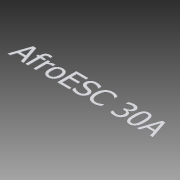
# Autodesk Inventor part: afro
Saved by Autodesk Inventor 2012 (Build 160160000, 160)
## iProperties
Created: 2014-07-18
Part Number: afro
Material: Default
Document SubType Name: Modeling
Designer: Anon
Density: 1 g/cm^3
Author: Anon
Autodesk Inventor part; units mm, degrees
ref_plane "YZ Plane" through (0, 0, 0) normal (1, 0, 0) x (0, 1, 0)
ref_plane "XZ Plane" through (0, 0, 0) normal (0, 1, 0) x (-1, 0, 0)
ref_plane "XY Plane" through (0, 0, 0) normal (0, 0, 1) x (1, 0, 0)
sketch "Sketch1" plane through (0, 0, 0) normal (0, 0, 1) x (1, 0, 0)
  line L0 (-5.9322, 2.9237) -> (28.5593, 2.9237) construction
  line L1 (28.5593, 2.9237) -> (28.5593, -13.2627) construction
  line L2 (28.5593, -13.2627) -> (-5.9322, -13.2627) construction
  line L3 (-5.9322, -13.2627) -> (-5.9322, 2.9237) construction
  line L4 (-5.9549, -0.755) -> (-4.775, 2.745)
  line L5 (-4.775, 2.745) -> (-4.2021, 2.745)
  line L6 (-4.2021, 2.745) -> (-3.0222, -0.755)
  line L7 (-3.0222, -0.755) -> (-3.5128, -0.755)
  line L8 (-3.5128, -0.755) -> (-3.8305, 0.2236)
  line L9 (-3.8305, 0.2236) -> (-5.1664, 0.2236)
  line L10 (-5.1664, 0.2236) -> (-5.4841, -0.755)
  line L11 (-5.4841, -0.755) -> (-5.9549, -0.755)
  line L12 (-3.9581, 0.6206) -> (-4.4999, 2.2685)
  line L13 (-4.4999, 2.2685) -> (-5.0388, 0.6206)
  line L14 (-5.0388, 0.6206) -> (-3.9581, 0.6206)
  line L15 (-1.3431, 2.4756) -> (-1.3658, 2.4756)
  spline S0 degree 2 poles (-1.3658, 2.4756) (-1.4253, 2.4983) (-1.6465, 2.538) (-1.7345, 2.538) knots 0 0 0 1 2 2 2
  spline S1 degree 2 poles (-1.7345, 2.538) (-2.0124, 2.538) (-2.2507, 2.2884) (-2.2507, 1.9594) knots 0 0 0 1 2 2 2
  line L16 (-2.2507, 1.9594) -> (-2.2507, 1.8715)
  line L17 (-2.2507, 1.8715) -> (-1.5189, 1.8715)
  line L18 (-1.5189, 1.8715) -> (-1.5189, 1.5056)
  line L19 (-1.5189, 1.5056) -> (-2.2365, 1.5056)
  line L20 (-2.2365, 1.5056) -> (-2.2365, -0.755)
  line L21 (-2.2365, -0.755) -> (-2.679, -0.755)
  line L22 (-2.679, -0.755) -> (-2.679, 1.5056)
  line L23 (-2.679, 1.5056) -> (-2.9768, 1.5056)
  line L24 (-2.9768, 1.5056) -> (-2.9768, 1.8715)
  line L25 (-2.9768, 1.8715) -> (-2.679, 1.8715)
  line L26 (-2.679, 1.8715) -> (-2.679, 1.9594)
  spline S2 degree 2 poles (-2.679, 1.9594) (-2.679, 2.4302) (-2.2223, 2.9237) (-1.7969, 2.9237) knots 0 0 0 1 2 2 2
  spline S3 degree 2 poles (-1.7969, 2.9237) (-1.6749, 2.9237) (-1.4395, 2.8982) (-1.3431, 2.8812) knots 0 0 0 1 2 2 2
  line L27 (-1.3431, 2.8812) -> (-1.3431, 2.4756)
  line L28 (0.1999, 1.3978) -> (0.1772, 1.3978)
  spline S4 degree 2 poles (0.1772, 1.3978) (0.1261, 1.412) (0.0155, 1.4177) (-0.0611, 1.4177) knots 0 0 0 1 2 2 2
  spline S5 degree 2 poles (-0.0611, 1.4177) (-0.2397, 1.4177) (-0.5914, 1.2617) (-0.7503, 1.1085) knots 0 0 0 1 2 2 2
  line L29 (-0.7503, 1.1085) -> (-0.7503, -0.755)
  line L30 (-0.7503, -0.755) -> (-1.1927, -0.755)
  line L31 (-1.1927, -0.755) -> (-1.1927, 1.8715)
  line L32 (-1.1927, 1.8715) -> (-0.7503, 1.8715)
  line L33 (-0.7503, 1.8715) -> (-0.7503, 1.48)
  spline S6 degree 2 poles (-0.7503, 1.48) (-0.5092, 1.6956) (-0.149, 1.8715) (0.0212, 1.8715) knots 0 0 0 1 2 2 2
  spline S7 degree 2 poles (0.0212, 1.8715) (0.0893, 1.8715) (0.1573, 1.8658) (0.1999, 1.8573) knots 0 0 0 1 2 2 2
  line L34 (0.1999, 1.8573) -> (0.1999, 1.3978)
  spline S8 degree 2 poles (2.7015, 0.5583) (2.7015, -0.1054) (2.0633, -0.8287) (1.5301, -0.8287) knots 0 0 0 1 2 2 2
  spline S9 degree 2 poles (1.5301, -0.8287) (0.9827, -0.8287) (0.3559, -0.0828) (0.3559, 0.5583) knots 0 0 0 1 2 2 2
  spline S10 degree 2 poles (0.3559, 0.5583) (0.3559, 1.2163) (1.0026, 1.9452) (1.5301, 1.9452) knots 0 0 0 1 2 2 2
  spline S11 degree 2 poles (1.5301, 1.9452) (2.0633, 1.9452) (2.7015, 1.2191) (2.7015, 0.5583) knots 0 0 0 1 2 2 2
  spline S12 degree 2 poles (2.2449, 0.5583) (2.2449, 1.0688) (1.8733, 1.5651) (1.5301, 1.5651) knots 0 0 0 1 2 2 2
  spline S13 degree 2 poles (1.5301, 1.5651) (1.1869, 1.5651) (0.8125, 1.0688) (0.8125, 0.5583) knots 0 0 0 1 2 2 2
  spline S14 degree 2 poles (0.8125, 0.5583) (0.8125, 0.0619) (1.1869, -0.4486) (1.5301, -0.4486) knots 0 0 0 1 2 2 2
  spline S15 degree 2 poles (1.5301, -0.4486) (1.8705, -0.4486) (2.2449, 0.0534) (2.2449, 0.5583) knots 0 0 0 1 2 2 2
  line L35 (3.1894, -0.755) -> (3.1894, 2.745)
  line L36 (3.1894, 2.745) -> (5.379, 2.745)
  line L37 (5.379, 2.745) -> (5.379, 2.3309)
  line L38 (5.379, 2.3309) -> (3.6545, 2.3309)
  line L39 (3.6545, 2.3309) -> (3.6545, 1.3723)
  line L40 (3.6545, 1.3723) -> (5.2627, 1.3723)
  line L41 (5.2627, 1.3723) -> (5.2627, 0.9582)
  line L42 (5.2627, 0.9582) -> (3.6545, 0.9582)
  line L43 (3.6545, 0.9582) -> (3.6545, -0.3409)
  line L44 (3.6545, -0.3409) -> (5.379, -0.3409)
  line L45 (5.379, -0.3409) -> (5.379, -0.755)
  line L46 (5.379, -0.755) -> (3.1894, -0.755)
  spline S16 degree 2 poles (6.8652, -0.8174) (6.4851, -0.8174) (5.9519, -0.6585) (5.7165, -0.5451) knots 0 0 0 1 2 2 2
  line L47 (5.7165, -0.5451) -> (5.7165, 0.0392)
  line L48 (5.7165, 0.0392) -> (5.7505, 0.0392)
  spline S17 degree 2 poles (5.7505, 0.0392) (5.9803, -0.1764) (6.5617, -0.4146) (6.8312, -0.4146) knots 0 0 0 1 2 2 2
  spline S18 degree 2 poles (6.8312, -0.4146) (7.2169, -0.4146) (7.6112, -0.0941) (7.6112, 0.1697) knots 0 0 0 1 2 2 2
  spline S19 degree 2 poles (7.6112, 0.1697) (7.6112, 0.3796) (7.4041, 0.6405) (7.18, 0.7057) knots 0 0 0 1 2 2 2
  spline S20 degree 2 poles (7.18, 0.7057) (7.0184, 0.7511) (6.7489, 0.8135) (6.5475, 0.8646) knots 0 0 0 1 2 2 2
  spline S21 degree 2 poles (6.5475, 0.8646) (6.366, 0.9128) (6.0795, 1.0574) (5.9689, 1.1737) knots 0 0 0 1 2 2 2
  spline S22 degree 2 poles (5.9689, 1.1737) (5.8612, 1.29) (5.742, 1.602) (5.742, 1.8062) knots 0 0 0 1 2 2 2
  spline S23 degree 2 poles (5.742, 1.8062) (5.742, 2.2317) (6.4057, 2.8074) (6.9191, 2.8074) knots 0 0 0 1 2 2 2
  spline S24 degree 2 poles (6.9191, 2.8074) (7.2141, 2.8074) (7.7359, 2.6912) (7.96, 2.5805) knots 0 0 0 1 2 2 2
  line L49 (7.96, 2.5805) -> (7.96, 2.0246)
  line L50 (7.96, 2.0246) -> (7.926, 2.0246)
  spline S25 degree 2 poles (7.926, 2.0246) (7.7586, 2.1778) (7.2368, 2.4047) (6.9503, 2.4047) knots 0 0 0 1 2 2 2
  spline S26 degree 2 poles (6.9503, 2.4047) (6.627, 2.4047) (6.227, 2.1012) (6.227, 1.8544) knots 0 0 0 1 2 2 2
  spline S27 degree 2 poles (6.227, 1.8544) (6.227, 1.6332) (6.4624, 1.3694) (6.6837, 1.3099) knots 0 0 0 1 2 2 2
  spline S28 degree 2 poles (6.6837, 1.3099) (6.8312, 1.2702) (7.2594, 1.1681) (7.4013, 1.1255) knots 0 0 0 1 2 2 2
  spline S29 degree 2 poles (7.4013, 1.1255) (7.7615, 1.0149) (8.0962, 0.5696) (8.0962, 0.2434) knots 0 0 0 1 2 2 2
  spline S30 degree 2 poles (8.0962, 0.2434) (8.0962, 0.0364) (7.9288, -0.3607) (7.7785, -0.4997) knots 0 0 0 1 2 2 2
  spline S31 degree 2 poles (7.7785, -0.4997) (7.6112, -0.6529) (7.1857, -0.8174) (6.8652, -0.8174) knots 0 0 0 1 2 2 2
  spline S32 degree 2 poles (9.9369, -0.8174) (9.5966, -0.8174) (9.0208, -0.5876) (8.8109, -0.3579) knots 0 0 0 1 2 2 2
  spline S33 degree 2 poles (8.8109, -0.3579) (8.601, -0.131) (8.3713, 0.5497) (8.3713, 0.9922) knots 0 0 0 1 2 2 2
  spline S34 degree 2 poles (8.3713, 0.9922) (8.3713, 1.4318) (8.5953, 2.0842) (8.8081, 2.3253) knots 0 0 0 1 2 2 2
  spline S35 degree 2 poles (8.8081, 2.3253) (9.018, 2.5607) (9.5909, 2.8074) (9.9454, 2.8074) knots 0 0 0 1 2 2 2
  spline S36 degree 2 poles (9.9454, 2.8074) (10.1213, 2.8074) (10.4304, 2.7564) (10.5609, 2.7167) knots 0 0 0 1 2 2 2
  spline S37 degree 2 poles (10.5609, 2.7167) (10.6744, 2.6798) (10.9098, 2.5749) (11.0261, 2.5125) knots 0 0 0 1 2 2 2
  line L51 (11.0261, 2.5125) -> (11.0261, 1.9509)
  line L52 (11.0261, 1.9509) -> (10.9892, 1.9509)
  spline S38 degree 2 poles (10.9892, 1.9509) (10.9268, 2.0076) (10.7339, 2.1664) (10.5949, 2.243) knots 0 0 0 1 2 2 2
  spline S39 degree 2 poles (10.5949, 2.243) (10.4616, 2.3168) (10.1468, 2.4104) (9.9426, 2.4104) knots 0 0 0 1 2 2 2
  spline S40 degree 2 poles (9.9426, 2.4104) (9.7185, 2.4104) (9.3186, 2.226) (9.1683, 2.0501) knots 0 0 0 1 2 2 2
  spline S41 degree 2 poles (9.1683, 2.0501) (9.0208, 1.8715) (8.8563, 1.3297) (8.8563, 0.9922) knots 0 0 0 1 2 2 2
  spline S42 degree 2 poles (8.8563, 0.9922) (8.8563, 0.632) (9.0293, 0.113) (9.1796, -0.0657) knots 0 0 0 1 2 2 2
  spline S43 degree 2 poles (9.1796, -0.0657) (9.3271, -0.2388) (9.7214, -0.4146) (9.9426, -0.4146) knots 0 0 0 1 2 2 2
  spline S44 degree 2 poles (9.9426, -0.4146) (10.144, -0.4146) (10.4872, -0.3153) (10.6205, -0.2416) knots 0 0 0 1 2 2 2
  spline S45 degree 2 poles (10.6205, -0.2416) (10.7481, -0.1678) (10.9381, -0.0147) (10.992, 0.0392) knots 0 0 0 1 2 2 2
  line L53 (10.992, 0.0392) -> (11.0261, 0.0392)
  line L54 (11.0261, 0.0392) -> (11.0261, -0.5167)
  spline S46 degree 2 poles (11.0261, -0.5167) (10.9098, -0.5706) (10.7056, -0.6699) (10.5609, -0.7153) knots 0 0 0 1 2 2 2
  spline S47 degree 2 poles (10.5609, -0.7153) (10.4077, -0.7663) (10.1468, -0.8174) (9.9369, -0.8174) knots 0 0 0 1 2 2 2
  spline S48 degree 2 poles (13.8085, 2.4132) (13.6808, 2.4132) (13.4284, 2.3508) (13.3065, 2.3026) knots 0 0 0 1 2 2 2
  spline S49 degree 2 poles (13.3065, 2.3026) (13.193, 2.2544) (13.0257, 2.1523) (12.9604, 2.1069) knots 0 0 0 1 2 2 2
  line L55 (12.9604, 2.1069) -> (12.9321, 2.1069)
  line L56 (12.9321, 2.1069) -> (12.9321, 2.6032)
  spline S50 degree 2 poles (12.9321, 2.6032) (13.0852, 2.6855) (13.6099, 2.8188) (13.8453, 2.8188) knots 0 0 0 1 2 2 2
  spline S51 degree 2 poles (13.8453, 2.8188) (14.0836, 2.8188) (14.4381, 2.7224) (14.5828, 2.6202) knots 0 0 0 1 2 2 2
  spline S52 degree 2 poles (14.5828, 2.6202) (14.7359, 2.5096) (14.8948, 2.1891) (14.8948, 1.9736) knots 0 0 0 1 2 2 2
  spline S53 degree 2 poles (14.8948, 1.9736) (14.8948, 1.6843) (14.5147, 1.2475) (14.2481, 1.1907) knots 0 0 0 1 2 2 2
  line L57 (14.2481, 1.1907) -> (14.2481, 1.1567)
  spline S54 degree 2 poles (14.2481, 1.1567) (14.3587, 1.134) (14.6112, 1.0319) (14.7189, 0.9298) knots 0 0 0 1 2 2 2
  spline S55 degree 2 poles (14.7189, 0.9298) (14.8267, 0.8305) (14.9629, 0.5129) (14.9629, 0.2831) knots 0 0 0 1 2 2 2
  spline S56 degree 2 poles (14.9629, 0.2831) (14.9629, 0.0477) (14.8012, -0.3522) (14.6537, -0.5054) knots 0 0 0 1 2 2 2
  spline S57 degree 2 poles (14.6537, -0.5054) (14.5005, -0.6642) (14.0666, -0.8287) (13.7915, -0.8287) knots 0 0 0 1 2 2 2
  spline S58 degree 2 poles (13.7915, -0.8287) (13.5277, -0.8287) (13.0115, -0.7011) (12.8356, -0.6131) knots 0 0 0 1 2 2 2
  line L58 (12.8356, -0.6131) -> (12.8356, -0.1168)
  line L59 (12.8356, -0.1168) -> (12.8697, -0.1168)
  spline S59 degree 2 poles (12.8697, -0.1168) (13.0171, -0.2246) (13.5163, -0.4231) (13.7631, -0.4231) knots 0 0 0 1 2 2 2
  spline S60 degree 2 poles (13.7631, -0.4231) (13.9077, -0.4231) (14.1971, -0.3323) (14.2935, -0.2274) knots 0 0 0 1 2 2 2
  spline S61 degree 2 poles (14.2935, -0.2274) (14.3871, -0.1225) (14.4864, 0.1271) (14.4864, 0.3172) knots 0 0 0 1 2 2 2
  spline S62 degree 2 poles (14.4864, 0.3172) (14.4864, 0.5072) (14.3757, 0.754) (14.2765, 0.8249) knots 0 0 0 1 2 2 2
  spline S63 degree 2 poles (14.2765, 0.8249) (14.1772, 0.8958) (13.9077, 0.9497) (13.7489, 0.9497) knots 0 0 0 1 2 2 2
  line L60 (13.7489, 0.9497) -> (13.5504, 0.9497)
  line L61 (13.5504, 0.9497) -> (13.5504, 1.3382)
  line L62 (13.5504, 1.3382) -> (13.7064, 1.3382)
  spline S64 degree 2 poles (13.7064, 1.3382) (14.0212, 1.3382) (14.4183, 1.6389) (14.4183, 1.9253) knots 0 0 0 1 2 2 2
  spline S65 degree 2 poles (14.4183, 1.9253) (14.4183, 2.0587) (14.3162, 2.2487) (14.2339, 2.3054) knots 0 0 0 1 2 2 2
  spline S66 degree 2 poles (14.2339, 2.3054) (14.146, 2.365) (13.9304, 2.4132) (13.8085, 2.4132) knots 0 0 0 1 2 2 2
  spline S67 degree 2 poles (17.6687, 0.995) (17.6687, 0.0534) (17.1213, -0.8287) (16.5512, -0.8287) knots 0 0 0 1 2 2 2
  spline S68 degree 2 poles (16.5512, -0.8287) (15.9726, -0.8287) (15.4308, 0.0704) (15.4308, 0.9922) knots 0 0 0 1 2 2 2
  spline S69 degree 2 poles (15.4308, 0.9922) (15.4308, 1.9395) (15.9783, 2.8159) (16.5512, 2.8159) knots 0 0 0 1 2 2 2
  spline S70 degree 2 poles (16.5512, 2.8159) (17.127, 2.8159) (17.6687, 1.9083) (17.6687, 0.995) knots 0 0 0 1 2 2 2
  spline S71 degree 2 poles (17.0674, -0.0714) (17.1355, 0.1016) (17.1922, 0.6348) (17.1922, 0.995) knots 0 0 0 1 2 2 2
  spline S72 degree 2 poles (17.1922, 0.995) (17.1922, 1.3553) (17.1355, 1.8856) (17.0646, 2.0643) knots 0 0 0 1 2 2 2
  spline S73 degree 2 poles (17.0646, 2.0643) (16.9936, 2.243) (16.7469, 2.4274) (16.5512, 2.4274) knots 0 0 0 1 2 2 2
  spline S74 degree 2 poles (16.5512, 2.4274) (16.3555, 2.4274) (16.103, 2.243) (16.0293, 2.0587) knots 0 0 0 1 2 2 2
  spline S75 degree 2 poles (16.0293, 2.0587) (15.9584, 1.88) (15.9073, 1.3354) (15.9073, 0.9922) knots 0 0 0 1 2 2 2
  spline S76 degree 2 poles (15.9073, 0.9922) (15.9073, 0.6235) (15.9527, 0.13) (16.0265, -0.0629) knots 0 0 0 1 2 2 2
  spline S77 degree 2 poles (16.0265, -0.0629) (16.0945, -0.2444) (16.347, -0.4401) (16.5512, -0.4401) knots 0 0 0 1 2 2 2
  spline S78 degree 2 poles (16.5512, -0.4401) (16.7441, -0.4401) (16.9965, -0.2558) (17.0674, -0.0714) knots 0 0 0 1 2 2 2
  line L63 (17.8389, -0.755) -> (19.0188, 2.745)
  line L64 (19.0188, 2.745) -> (19.5917, 2.745)
  line L65 (19.5917, 2.745) -> (20.7716, -0.755)
  line L66 (20.7716, -0.755) -> (20.2809, -0.755)
  line L67 (20.2809, -0.755) -> (19.9633, 0.2236)
  line L68 (19.9633, 0.2236) -> (18.6274, 0.2236)
  line L69 (18.6274, 0.2236) -> (18.3097, -0.755)
  line L70 (18.3097, -0.755) -> (17.8389, -0.755)
  line L71 (19.8356, 0.6206) -> (19.2939, 2.2685)
  line L72 (19.2939, 2.2685) -> (18.755, 0.6206)
  line L73 (18.755, 0.6206) -> (19.8356, 0.6206)
  point P0 (0, 0)
  constraints: 2 other
extrude "Extrusion1" add sketch "Sketch1" along normal blind 0.1
body "Solid1"
